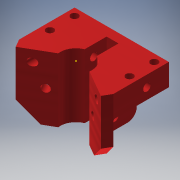
# Autodesk Inventor part: Linear_pipe
Saved by Autodesk Inventor 2016 SP2 (Build 200236200, 236)
## iProperties
Created: 2017-08-14
Part Number: Linear_pipe
Material: ABS Plastic
Document SubType Name: Modeling
Designer: Admin
Density: 1.06 g/cm^3
Appearance: Smooth - White
Mass: 189.673 g
Surface Area: 440.519 cm^2
Volume: 178.937 cm^3
Author: Admin
Autodesk Inventor part; units mm, degrees
ref_plane "YZ Plane" through (0, 0, 0) normal (1, 0, 0) x (0, 1, 0)
ref_plane "XZ Plane" through (0, 0, 0) normal (0, 1, 0) x (-1, 0, 0)
ref_plane "XY Plane" through (0, 0, 0) normal (0, 0, 1) x (1, 0, 0)
sketch "Sketch1" plane through (0, 0, 0) normal (0, 0, 1) x (1, 0, 0)
  circle A0 centre (0, 0) radius 15 construction
  circle A1 centre (0, 0) radius 26 construction
  line L0 (3.5, 37) -> (-3.5, 37) construction
  line L1 (-3.5, 37) -> (-3.5, 15) construction
  line L2 (-3.5, 15) -> (3.5, 15) construction
  line L3 (3.5, 15) -> (3.5, 37) construction
  line L4 (3.5, 37) -> (-3.5, 15) construction
  line L5 (-3.5, 37) -> (3.5, 15) construction
  line L6 (-6.5, 16) -> (-6.5, 40) construction
  line L7 (-6.5, 40) -> (6.5, 40) construction
  line L8 (6.5, 40) -> (6.5, 16) construction
  circle A2 centre (0, 0) radius 17.2699 construction
  line L9 (-16.5, 16) -> (-16.5, 50) construction
  line L10 (-16.5, 50) -> (16.5, 50) construction
  line L11 (16.5, 50) -> (16.5, 16) construction
  circle A3 centre (0, 0) radius 23 construction
  line L12 (-25, 26) -> (25, 26) construction
  line L13 (-25, 30) -> (25, 30) construction
  line L14 (-25, 22) -> (25, 22) construction
  line L15 (-35.0513, -39.2894) -> (-51.5513, -10.7106) construction
  line L16 (-31.391, -25.6292) -> (-37.891, -14.3708) construction
  line L17 (-5.6064, -22.2894) -> (-35.0513, -39.2894) construction
  line L18 (-51.5513, -10.7106) -> (-22.1064, 6.2894) construction
  line L19 (-37.891, -14.3708) -> (-17.1064, -2.3708) construction
  line L20 (-10.6064, -13.6292) -> (-31.391, -25.6292) construction
  line L21 (-30.2929, -21.5311) -> (-11.2404, -10.5311) construction
  line L22 (-11.2404, -10.5311) -> (-14.7404, -4.4689) construction
  line L23 (-14.7404, -4.4689) -> (-33.7929, -15.4689) construction
  line L24 (-33.7929, -15.4689) -> (-11.2404, -10.5311) construction
  line L25 (-30.2929, -21.5311) -> (-14.7404, -4.4689) construction
  line L26 (-33.7929, -15.4689) -> (-30.2929, -21.5311) construction
  line L27 (-13.4808, -36.6506) -> (-38.4808, 6.6506) construction
  line L28 (-10.0167, -34.6506) -> (-35.0167, 8.6506) construction
  line L29 (-6.5526, -32.6506) -> (-31.5526, 10.6506) construction
  line L30 (51.5513, -10.7106) -> (35.0513, -39.2894) construction
  line L31 (37.891, -14.3708) -> (31.391, -25.6292) construction
  line L32 (22.1064, 6.2894) -> (51.5513, -10.7106) construction
  line L33 (35.0513, -39.2894) -> (5.6064, -22.2894) construction
  line L34 (31.391, -25.6292) -> (10.6064, -13.6292) construction
  line L35 (17.1064, -2.3708) -> (37.891, -14.3708) construction
  line L36 (33.7929, -15.4689) -> (14.7404, -4.4689) construction
  line L37 (14.7404, -4.4689) -> (11.2404, -10.5311) construction
  line L38 (11.2404, -10.5311) -> (30.2929, -21.5311) construction
  line L39 (30.2929, -21.5311) -> (14.7404, -4.4689) construction
  line L40 (33.7929, -15.4689) -> (11.2404, -10.5311) construction
  line L41 (30.2929, -21.5311) -> (33.7929, -15.4689) construction
  line L42 (38.4808, 6.6506) -> (13.4808, -36.6506) construction
  line L43 (35.0167, 8.6506) -> (10.0167, -34.6506) construction
  line L44 (31.5526, 10.6506) -> (6.5526, -32.6506) construction
  line L45 (-16.5, 16.0234) -> (-16.5, 50)
  line L46 (-16.5, 50) -> (16.5, 50)
  line L47 (16.5, 50) -> (16.5, 16.0234)
  line L48 (-6.5, 16) -> (-6.5, 40)
  line L49 (-6.5, 40) -> (6.5, 40)
  line L50 (6.5, 40) -> (6.5, 16)
  line L51 (-22.1267, 6.2777) -> (-51.5513, -10.7106)
  line L52 (-51.5513, -10.7106) -> (-46.5513, -19.3708)
  line L53 (-46.5513, -19.3708) -> (-17.1064, -2.3708)
  line L54 (46.5513, -19.3708) -> (51.5513, -10.7106)
  line L55 (51.5513, -10.7106) -> (22.1267, 6.2777)
  line L56 (17.1064, -2.3708) -> (46.5513, -19.3708)
  line L57 (37.891, -14.3708) -> (31.391, -25.6292)
  arc A4 (-6.5, 16) -> (-17.1064, -2.3708) centre (0, 0) ccw
  arc A5 (-16.5, 16.0234) -> (-22.1267, 6.2777) centre (0, 0) ccw
  arc A6 (17.1064, -2.3708) -> (6.5, 16) centre (0, 0) ccw
  arc A7 (22.1267, 6.2777) -> (16.5, 16.0234) centre (0, 0) ccw
  point P0 (0, 26)
  point P1 (0, 26)
  point P2 (0, 26)
  point P3 (0, 30)
  point P4 (0, 22)
  point P5 (-25.9808, -15)
  point P6 (-22.5167, -13)
  point P7 (-22.5167, -13)
  point P8 (-22.5167, -13)
  point P9 (-5.6267, -22.3011)
  point P10 (-19.0526, -11)
  point P11 (25.9808, -15)
  point P12 (22.5167, -13)
  point P13 (22.5167, -13)
  point P14 (22.5167, -13)
  point P15 (19.0526, -11)
  dimension "d1" = 52
  dimension "d0" = 30
  dimension "d2" = 7
  dimension "d4" = 3
  dimension "d5" = 3
  dimension "d6" = 3
  dimension "d7" = 16
  dimension "d8" = 10
  dimension "d9" = 10
  dimension "d11" = 10
  dimension "d12" = 3
  dimension "d13" = 50
  dimension "d14" = 4
  dimension "d15" = 4
  dimension "d16" = 50
  dimension "d17" = 50
  dimension "d20" = 360
  constraints: 116 end point, 11 midpoint, 11 point on circle, 8 collinear, 8 perpendicular, 8 point on line, 7 parallel, 6 centre point, 4 coincident, 4 horizontal, 4 vertical alignment, 3 horizontal alignment, 2 concentric, 1 tangent, 125 other
  measures "d0" diameter of A0
  measures "d2" distance of L0.start L0.end
  measures "d4" distance between parallel lines of L0 L7
  measures "d5" distance between parallel lines of L6 L1
  measures "d6" distance between parallel lines of L8 L3
  measures "d7" vertical distance of A0.centre L6.start
  measures "d8" distance between parallel lines of L9 L6
  measures "d9" distance between parallel lines of L11 L8
  measures "d11" distance between parallel lines of L10 L7
  measures "d13" distance of L12.start L12.end
  measures "d14" distance of L12.start L13.start
  measures "d15" distance between parallel lines of L12 L14
  measures "d16" distance of L14.end L14.start
  measures "d17" distance of L13.end L13.start
extrude "Extrusion3" add sketch "Sketch1" along normal blind 70
sketch "Sketch6" plane through (16.5, 16.0234, 0) normal (1, 0, 0) x (0, 0, -1)
  line L0 (0, 9.9766) -> (-71.7893, 9.9766) construction
  line L1 (-70, 0) -> (-70, 33.9766) construction
  point P0 (0, -16.0234)
  point P1 (0, 9.9766)
  point P2 (-58, 9.9766)
  point P3 (-12, 9.9766)
  dimension "d46" = 12
  dimension "d47" = 12
  constraints: 2 end point, 2 point on line, 1 perpendicular
  measures "d46" distance of point (0, 9.977) point (-12, 9.977)
  measures "d47" distance from line of L1 point (-58, 9.977)
sketch "Sketch7" plane through (0, 0, 70) normal (0, 0, 1) x (1, 0, 0)
  line L0 (-22.1267, 6.2777) -> (-51.5513, -10.7106) projected
  line L1 (-51.5513, -10.7106) -> (-51.5513, 50)
  line L2 (-51.5513, 50) -> (-16.5, 50)
  line L3 (16.5, 16.0234) -> (16.5, 50) projected
  line L4 (16.5, 50) -> (51.5513, 50)
  line L5 (51.5513, 50) -> (51.5513, -10.7106)
  arc A0 (-16.5, 16.0234) -> (-22.1267, 6.2777) centre (0, 0) ccw projected
  line L6 (-16.5, 50) -> (-16.5, 16.0234) projected
  arc A1 (22.1267, 6.2777) -> (16.5, 16.0234) centre (0, 0) ccw projected
  line L7 (51.5513, -10.7106) -> (22.1267, 6.2777) projected
  line L8 (51.5513, 50) -> (51.5513, -10.7106)
  point P0 (0, 0)
  point P1 (16.5, 26)
  constraints: 10 end point, 2 perpendicular, 2 vertical, 1 point on line
extrude "Extrusion5" add sketch "Sketch7" against normal blind 24
hole "Hole3" at (16.5, 26, 58) at (16.5, 26, 12) direction (-1, 0, 0) diameter 8.2 end through all
hole "Hole4" at (-51.5513, 26, 58) direction (1, 0, 0) diameter 8.2 end through all
sketch "Sketch10" plane through (-22.1267, 6.2777, 46) normal (-0.5, 0.866, 0) x (0.866, 0.5, 0)
  line L0 (-9.9766, 46) -> (-9.9766, -2.7834) construction
  line L1 (-33.9766, 0) -> (0, 0) construction
  line L2 (-33.9766, 46) -> (-33.9766, -24) construction
  line L3 (-33.9766, 11) -> (0, 11) construction
  line L4 (0, 46) -> (0, 0) construction
  point P0 (16.0234, 46)
  point P1 (-9.9766, 46)
  point P2 (-9.9766, 11)
  constraints: 4 end point, 3 point on line, 1 horizontal, 1 midpoint, 1 perpendicular
hole "Hole5" at (-30.7667, 1.2894, 35) direction (0.5, -0.866, 0) diameter 8.2 end through all
sketch "Sketch11" plane through (51.5513, -10.7106, 46) normal (0.5, 0.866, 0) x (0.866, -0.5, 0)
  line L0 (-24, 46) -> (-24, 0) construction
  line L1 (-33.9766, 0) -> (0, 0) construction
  line L2 (0, 46) -> (0, -24) construction
  line L3 (0, 11) -> (-34, 11) construction
  line L4 (-34, 46) -> (-34, -24) construction
  point P0 (-50, 46)
  point P1 (-24, 11)
  constraints: 4 end point, 3 point on line, 2 midpoint, 1 vertical
hole "Hole6" at (30.7667, 1.2894, 35) direction (-0.5, -0.866, 0) diameter 8.2 end through all
fillet "Fillet2" radius 2 10 edges at (-36.839, -2.2164, 46) (-19.9186, 11.5, 46) (-16.5, 33.0117, 46) (-16.5, 16.0234, 23) (-22.1267, 6.2777, 23) (16.5, 16.0234, 23) (22.1267, 6.2777, 23) (16.5, 33.0117, 46) (19.9186, 11.5, 46) (36.839, -2.2164, 46)
fillet "Fillet3" radius 10 1 edges at (0, 50, 0)
chamfer "Chamfer1" distance 20 angle 45 2 edges at (49.0513, -15.0407, 0) (-49.0513, -15.0407, 0)
sketch "Sketch12" plane through (-51.5513, 50, 70) normal (0, 1, 0) x (1, 0, 0)
  line L0 (0, 0) -> (0, 24) construction
  line L1 (0, 12) -> (103.1025, 12) construction
  line L2 (103.1025, 0) -> (103.1025, 24) construction
  line L3 (0, 24) -> (33.0513, 24) construction
  line L4 (16.5256, 24) -> (16.5256, 0) construction
  line L5 (5, 0) -> (34.4449, 0) construction
  line L6 (70.0513, 24) -> (103.1025, 24) construction
  line L7 (86.5769, 24) -> (86.5769, 0) construction
  line L8 (103.1025, 0) -> (0, 0) construction
  point P0 (51.5513, 70)
  point P1 (86.5769, 12)
  point P2 (16.5256, 12)
  constraints: 6 end point, 6 midpoint, 2 point on line, 2 vertical
hole "Hole7" at (35.0256, 50, 58) at (-35.0256, 50, 58) direction (0, -1, 0) diameter 8.2 end through all
sketch "Sketch13" plane through (0, 0, 70) normal (0, 0, 1) x (1, 0, 0)
  line L0 (51.5513, 50) -> (-51.5513, 50) construction
  line L1 (-43.5513, 50) -> (-43.5513, -5) construction
  line L2 (0, 50) -> (0, -7.7688) construction
  point P0 (0, 0)
  point P1 (-43.5513, 42)
  point P2 (-43.5513, 15)
  point P3 (-43.5513, 42)
  point P4 (-43.5513, 15)
  point P5 (43.5513, 42)
  point P6 (43.5513, 15)
  point P7 (43.5513, 42)
  point P8 (43.5513, 15)
  dimension "d95" = 8
  dimension "d96" = 8
  dimension "d97" = 35
  constraints: 4 coincident, 4 end point, 4 symmetric about line, 3 point on line, 2 vertical, 1 midpoint
  measures "d95" distance of L0.end L1.start
  measures "d96" horizontal distance of L0.end point (-43.551, 42)
  measures "d97" vertical distance of L0.end point (-43.551, 15)
hole "Hole8" at (-43.5513, 42, 70) at (-43.5513, 15, 70) at (43.5513, 42, 70) at (43.5513, 15, 70) direction (0, 0, -1) diameter 8.2 end through all
sketch "Sketch14" plane through (0, 0, 70) normal (0, 0, 1) x (1, 0, 0)
  point P0 (0, 0)
sketch "Sketch15" plane through (0, 0, 70) normal (0, 0, 1) x (1, 0, 0)
  line L0 (-51.5513, 50) -> (-51.5513, -10.7106) projected
  line L1 (51.5513, -10.7106) -> (51.5513, 50) projected
  line L2 (-51.5513, -0.3388) -> (51.5513, -0.3388)
  line L3 (51.5513, -0.3388) -> (51.5513, -25.3388)
  line L4 (51.5513, -25.3388) -> (-51.5513, -25.3388)
  line L5 (-51.5513, -25.3388) -> (-51.5513, -0.3388)
  point P0 (0, 0)
  dimension "d105" = 25
  constraints: 8 end point, 2 parallel, 1 horizontal, 1 perpendicular, 1 point on line
  measures "d105" distance of L2.end L3.end
extrude "Extrusion6" cut sketch "Sketch15" against normal blind 22
equation "\"d5\" = d4"
equation "\"d6\" = d4"
equation "\"d9\" = d8"
equation "\"d15\" = d14"
equation "\"d16\" = d13"
equation "\"d17\" = d16"
equation "\"d46\" = d47"
equation "\"d50\" = 2 * d47"
body "Solid2"
